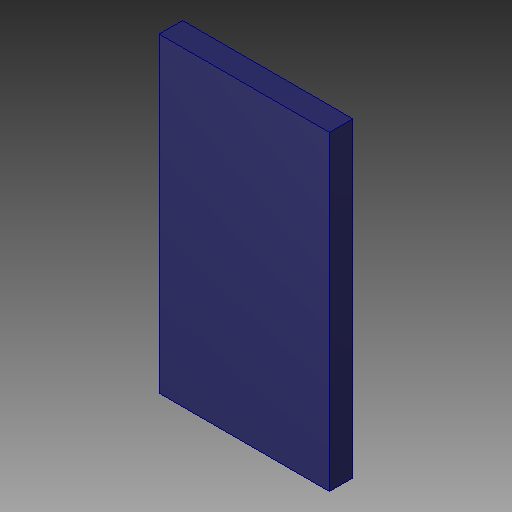
# Autodesk Inventor part: SCHALTER
Saved by Autodesk Inventor 2017 (Build 210142000, 142)
## iProperties
Created: 2019-06-13
Part Number: SCHALTER
Material: Generic
Document SubType Name: Modeling
Designer: Marc
Density: 1 g/cm^3
Appearance: SCHALTER, SCHALTER
Author: Marc
Autodesk Inventor part; units mm, degrees
ref_plane "YZ Plane" through (0, 0, 0) normal (1, 0, 0) x (0, 1, 0)
ref_plane "XZ Plane" through (0, 0, 0) normal (0, 1, 0) x (-1, 0, 0)
ref_plane "XY Plane" through (0, 0, 0) normal (0, 0, 1) x (1, 0, 0)
sketch "SCHALTER, SCHALTER_68" plane through (0, 0, 0) normal (0, 0, 1) x (1, 0, 0)
  line L0 (-0.0635, 0.0635) -> (7.2, 0.0635)
  line L1 (7.2, 0.0635) -> (7.2, -13.2)
  line L2 (7.2, -13.2) -> (-0.0635, -13.2)
  line L3 (-0.0635, -13.2) -> (-0.0635, 0.0635)
  constraints: 8 end point
extrude "Extrusion1" add sketch "SCHALTER, SCHALTER_68" along normal blind 1
body "Solid1"
